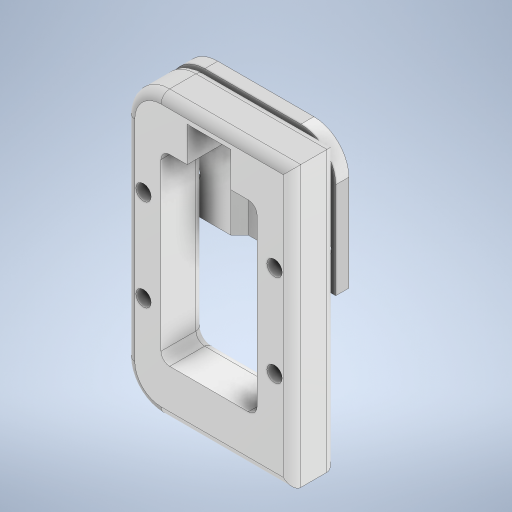
# Autodesk Inventor part: CoxaLeft
Saved by Autodesk Inventor 2024 (Build 280153000, 153)
## iProperties
Created: 2026-01-13
Part Number: CoxaLeft
Material: Generic
Document SubType Name: Modeling
Designer: Liam
Density: 1 g/cm^3
Appearance: Default
Author: Liam
Autodesk Inventor part; units mm, degrees
ref_plane "YZ Plane" through (0, 0, 0) normal (1, 0, 0) x (0, 1, 0)
ref_plane "XZ Plane" through (0, 0, 0) normal (0, 1, 0) x (-1, 0, 0)
ref_plane "XY Plane" through (0, 0, 0) normal (0, 0, 1) x (1, 0, 0)
sketch "Sketch1" plane through (0, 0, 0) normal (0, 0, 1) x (1, 0, 0)
  line L0 (0, 0) -> (22, 0)
  line L1 (22, 0) -> (22, 42)
  line L2 (22, 42) -> (0, 42)
  line L3 (0, 42) -> (0, 0)
  line L4 (-8, 50) -> (30, 50) construction
  line L5 (30, 50) -> (30, -8)
  line L6 (30, -8) -> (-8, -8)
  line L7 (-8, -8) -> (-8, 50)
  line L8 (0, 21) -> (22, 21) construction
  line L9 (11, 0) -> (11, 42) construction
  circle A0 centre (26, 10.5) radius 1.75
  circle A1 centre (26, 31.5) radius 1.75
  circle A2 centre (-4, 10.5) radius 1.75
  circle A3 centre (-4, 31.5) radius 1.75
  line L10 (0, 50) -> (22, 50)
  line L11 (22, 42) -> (0, 42)
  line L12 (0, 0) -> (22, 0)
  line L13 (22, -8) -> (0, -8)
  line L14 (5.4779, 42) -> (18.0265, 42)
  line L15 (5.4779, 0) -> (19.7232, 0)
  line L16 (-8, 50) -> (30, 50)
  line L17 (30, 50) -> (30, 53)
  line L18 (30, 53) -> (-8, 53)
  line L19 (-8, 53) -> (-8, 50)
  line L20 (-8, -8) -> (30, -8)
  line L21 (30, -8) -> (30, -11)
  line L22 (30, -11) -> (-8, -11)
  line L23 (-8, -11) -> (-8, -8)
  line L24 (16, 42) -> (6, 42)
  line L25 (6, 42) -> (6, 50)
  line L26 (6, 50) -> (16, 50)
  line L27 (16, 50) -> (16, 42)
  line L28 (16, 50) -> (6, 50)
  line L29 (6, 50) -> (6, 53)
  line L30 (6, 53) -> (16, 53)
  line L31 (16, 53) -> (16, 50)
  point P0 (6, 42)
  dimension "d0" = 42
  dimension "d2" = 8
  dimension "d3" = 3.5
  dimension "d4" = 10.5
  dimension "d5" = 4
  dimension "d6" = 8
  dimension "d15" = 22
  dimension "d18" = 3
  dimension "d19" = 38
  dimension "d20" = 38
  dimension "d21" = 3
  dimension "d63" = 10
  dimension "d64" = 5
  dimension "d65" = 8
  dimension "d72" = 10
  constraints: 64 end point, 14 parallel, 9 horizontal, 6 perpendicular, 6 point on line, 4 centre point, 4 midpoint, 3 symmetric about line, 6 other
  measures "d0" distance of L0.end L1.end
  measures "d2" distance between parallel lines of L4 L2
  measures "d3" diameter of A0
  measures "d4" distance from line of A0.centre L8
  measures "d5" distance from line of L1 A0.centre
  measures "d6" distance of L11.end L10.start
  measures "d15" distance of L1.end L2.end
  measures "d18" distance between parallel lines of L18 L4
  measures "d19" distance between parallel lines of L19 L17
  measures "d20" distance of L21.end L22.end
  measures "d21" distance of L20.end L21.end
  measures "d63" distance of L25.end L26.end
  measures "d64" distance between parallel lines of L25 L9
  measures "d65" distance of L24.end L25.end
  measures "d72" distance between parallel lines of L29 L31
extrude "Extrusion1" add sketch "Sketch1" along normal blind 10 contours L0 L1 L2 L27 L10 L16 L5 L6 L7 L25 L3 | L29 L18 L31 L10 | L10 L16 L19 L18 L29 | L31 L18 L17 L16 L10 | L6 L21 L22 L23
fillet "Fillet1" radius 8 2 edges at (-8, 53, 5) (-8, -11, 5)
fillet "Fillet2" radius 2 4 edges at (0, 42, 5) (0, 0, 5) (22, 0, 5) (22, 42, 5)
fillet "Fillet3" radius 2 15 edges at (30, 21, 0) (15, -11, 0) (15, 53, 0) (0.5858, 41.4142, 0) (18, 42, 0) (4, 42, 0) (21.4142, 41.4142, 0) (22, 21, 0) (21.4142, 0.5858, 0) (11, 0, 0) (0.5858, 0.5858, 0) (0, 21, 0) (30, 21, 10) (15, -11, 10) (15, 53, 10)
sketch "Sketch2" plane through (0, 0, 0) normal (0, 0, -1) x (-1, 0, 0)
  circle A0 centre (-11, 31) radius 5
  line L0 (-14, 34) -> (-8, 34)
  line L1 (-8, 34) -> (-8, 28)
  line L2 (-8, 28) -> (-14, 28)
  line L3 (-14, 28) -> (-14, 34)
  line L4 (-14, 34) -> (-8, 28) construction
  line L5 (-8, 34) -> (-14, 28) construction
  line L6 (-17, 37) -> (-5, 37)
  line L7 (-5, 37) -> (-5, 25)
  line L8 (-5, 25) -> (-17, 25)
  line L9 (-17, 25) -> (-17, 37)
  line L10 (-17, 37) -> (-5, 25) construction
  line L11 (-5, 37) -> (-17, 25) construction
  circle A1 centre (-11, 31) radius 2.5
  circle A2 centre (-26, 31.5) radius 1.75 projected
  circle A3 centre (-26, 31.5) radius 3
  circle A4 centre (4, 31.5) radius 1.75 projected
  circle A5 centre (4, 31.5) radius 3
  line L12 (8, 45) -> (8, -3) projected
  line L13 (-30, 53) -> (8, 53)
  line L14 (8, 53) -> (8, 23)
  line L15 (8, 23) -> (-30, 23)
  line L16 (-30, 23) -> (-30, 53)
  line L17 (-6, 50) -> (-16, 50) projected
  line L18 (-16, 50) -> (-6, 50)
  line L19 (-6, 50) -> (-6, 23)
  line L20 (-6, 23) -> (-16, 23)
  line L21 (-16, 23) -> (-16, 50)
  point P0 (0, 0)
  point P1 (8, 45)
  point P2 (-6, 25)
  point P3 (-6, 37)
  dimension "d28" = 10
  dimension "d31" = 6
  dimension "d32" = 6
  dimension "d33" = 12
  dimension "d34" = 12
  dimension "d35" = 5
  dimension "d56" = 6
  dimension "d57" = 6
  dimension "d59" = 30
  dimension "d60" = 22
  dimension "d61" = 38
  dimension "d62" = 19
  dimension "d66" = 10
  constraints: 40 end point, 8 parallel, 4 centre point, 4 horizontal, 4 midpoint, 4 perpendicular, 3 coincident, 2 point on line
  measures "d28" diameter of A0
  measures "d31" distance of L0.start L0.end
  measures "d32" distance of L0.end L1.end
  measures "d33" distance of L6.end L7.end
  measures "d34" distance of L6.start L6.end
  measures "d35" diameter of A1
  measures "d56" diameter of A3
  measures "d57" diameter of A5
  measures "d59" distance between parallel lines of L15 L13
  measures "d60" distance from line of L13 A0.centre
  measures "d61" distance of L14.end L15.end
  measures "d62" distance from line of L16 A0.centre
  measures "d66" distance between parallel lines of L19 L21
extrude "Extrusion3" add sketch "Sketch2" along normal blind 3 separate body contours L19 L17 L21 L6 L9 L8 L15 L16 L13 L14 L12 L7 | L6 L21 L17 L19 | L19 L15 L21 L8
extrude "Extrusion4" add sketch "Sketch2" along normal blind 3.5 contours A0 | L19 L8 L21 A0 | A0 L21 L6 L19 | L19 L6 L7 L8 | L21 L8 L9 L6 | L0 L1 L2 L3 | A1 bodies 2
extrude "Extrusion5" add sketch "Sketch2" along normal blind 11.5 contours A0 bodies 2
extrude "Extrusion6" add sketch "Sketch2" along normal blind 9.5 contours L0 L1 L2 L3 bodies 2
extrude "Extrusion7" add sketch "Sketch2" along normal blind 4.5 contours A1 bodies 2
fillet "Fillet4" radius 8 2 edges at (30, 53, -1.5) (-8, 53, -1.5)
extrude "Extrusion10" cut sketch "Sketch2" along normal blind 2 contours A0 | L19 L8 L21 A0 | A0 L21 L6 L19 | L6 L21 L17 L19 | L19 L15 L21 L8 | L0 L1 L2 L3 | A1 bodies 2
chamfer "Chamfer1" distance 2 angle 45 2 edges at (6, 36.5, -2) (16, 36.5, -2)
equation "\"d0\" = MOUNT_LENGTH"
equation "\"d2\" = MOUNT_THICKNESS"
equation "\"d3\" = ThroughDiameter"
equation "\"d4\" = 0.25 * MOUNT_LENGTH"
equation "\"d5\" = 0.5 * MOUNT_THICKNESS"
equation "\"d15\" = MOUNT_WIDTH"
equation "\"d18\" = -0.5 * MOUNT_LENGTH + 0.5 * COXA_JOINT_LENGTH"
equation "\"d19\" = MOUNT_WIDTH + 2 * MOUNT_THICKNESS"
equation "\"d20\" = MOUNT_WIDTH + 2 * MOUNT_THICKNESS"
equation "\"d21\" = -0.5 * MOUNT_LENGTH + 0.5 * COXA_JOINT_LENGTH"
equation "\"d64\" = 0.5 * d63"
equation "\"d58\" = OUTER_FILLET"
equation "\"d13\" = INNER_FILLET"
equation "\"d25\" = INNER_FILLET"
equation "\"d28\" = PIVOT_DIAMETER"
equation "\"d34\" = PIVOT_SQUARE"
equation "\"d35\" = HOLE_DIAMETER"
equation "\"d60\" = 0.5 * COXA_JOINT_LENGTH - 0.5 * MOUNT_LENGTH + TOP_TO_PIVOT"
equation "\"d62\" = 0.5 * d61"
equation "\"d38\" = PIVOT_PLATE_HEIGHT"
equation "\"d40\" = PIVOT_HEIGHT + PIVOT_PLATE_HEIGHT"
equation "\"d42\" = PIVOT_HEIGHT + PIVOT_PLATE_HEIGHT - PIVOT_DEPTH"
equation "\"d46\" = OUTER_FILLET"
equation "\"ThroughDiameter\" = 3.5"
equation "\"MOUNT_LENGTH\" = 42"
equation "\"MOUNT_THICKNESS\" = 8"
equation "\"MOUNT_WIDTH\" = 22"
equation "\"COXA_JOINT_LENGTH\" = 48"
equation "\"OUTER_FILLET\" = 8"
equation "\"INNER_FILLET\" = 2"
equation "\"PIVOT_DIAMETER\" = 10"
equation "\"PIVOT_SQUARE\" = 12"
equation "\"HOLE_DIAMETER\" = 5"
equation "\"TOP_TO_PIVOT\" = 19"
equation "\"PIVOT_PLATE_HEIGHT\" = 3.5"
equation "\"PIVOT_HEIGHT\" = 8"
equation "\"PIVOT_DEPTH\" = 2"
body "Solid1"
body "Solid2"
